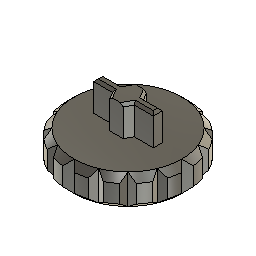
Better screw tool v4 (Autodesk Fusion 360 design; units mm, degrees)
Autodesk Fusion 360 part; units mm, degrees
note: some values were not read from the file. Set by a fixed rule: which sketch regions a step uses.
sketch "Sketch2" plane through (0, 0, 0) normal (0, 0, 1) x (1, 0, 0)
  circle A0 centre (0, 0) radius 10
  constraint coincident A0.centre origin
extrude "Extrude1" add sketch "Sketch2" along normal blind 5
chamfer "Chamfer1" distance 1 angle 45 2 edges at (-9.3233, -3.6162, 5) (-9.3233, -3.6162, 0)
sketch "Sketch3" plane through (0, 0, 5) normal (0, 0, 1) x (-1, 0, 0)
  circle A0 centre (0, 0) radius 9
  line L0 (1, -10) -> (0, -9)
  line L1 (1, -10) -> (2.4142, -10) construction
  line L2 (0, -9) -> (-1, -10)
  line L3 (-1, -10) -> (1, -10)
  dimension "d4" = 135
  constraint horizontal L1
  constraint coincident A0 L0.end
  constraint perpendicular L0 L2
  constraint parallel L1 L3
  measures "d4" angle of L0 L1
extrude "Extrude2" cut sketch "Sketch3" against normal blind 5 contours L0 L2 L3
pattern_circular "C-Pattern1" count 16 over 360 about axis through (0, 0, 1.75) along (0, 0, 1) of "Extrude2"
sketch "Sketch4" plane through (0, 0, 5) normal (0, 0, 1) x (-1, 0, 0)
  arc A0 (-3.4442, -8.3149) -> (0, -9) centre (0, 0) ccw
  arc A1 (0, -9) -> (3.4442, -8.3149) centre (0, 0) ccw
  arc A2 (3.4442, -8.3149) -> (6.364, -6.364) centre (0, 0) ccw
  arc A3 (6.364, -6.364) -> (8.3149, -3.4442) centre (0, 0) ccw
  arc A4 (8.3149, -3.4442) -> (9, 0) centre (0, 0) ccw
  arc A5 (9, 0) -> (8.3149, 3.4442) centre (0, 0) ccw
  arc A6 (8.3149, 3.4442) -> (6.364, 6.364) centre (0, 0) ccw
  arc A7 (6.364, 6.364) -> (3.4442, 8.3149) centre (0, 0) ccw
  arc A8 (3.4442, 8.3149) -> (0, 9) centre (0, 0) ccw
  arc A9 (0, 9) -> (-3.4442, 8.3149) centre (0, 0) ccw
  arc A10 (-3.4442, 8.3149) -> (-6.364, 6.364) centre (0, 0) ccw
  arc A11 (-6.364, 6.364) -> (-8.3149, 3.4442) centre (0, 0) ccw
  arc A12 (-8.3149, 3.4442) -> (-9, 0) centre (0, 0) ccw
  arc A13 (-9, 0) -> (-8.3149, -3.4442) centre (0, 0) ccw
  arc A14 (-8.3149, -3.4442) -> (-6.364, -6.364) centre (0, 0) ccw
  arc A15 (-6.364, -6.364) -> (-3.4442, -8.3149) centre (0, 0) ccw
  line L0 (5, 0.75) -> (-5, 0.75)
  line L1 (-5, 0.75) -> (-5, -0.75)
  line L2 (-5, -0.75) -> (5, -0.75)
  line L3 (5, -0.75) -> (5, 0.75)
  line L4 (5, 0.75) -> (-5, -0.75) construction
  line L5 (-5, 0.75) -> (5, -0.75) construction
  line L6 (-1.1258, -1.95) -> (1.1258, -1.95)
  line L7 (1.1258, -1.95) -> (2.2517, 0)
  line L8 (2.2517, 0) -> (1.1258, 1.95)
  line L9 (1.1258, 1.95) -> (-1.1258, 1.95)
  line L10 (-1.1258, 1.95) -> (-2.2517, 0)
  line L11 (-2.2517, 0) -> (-1.1258, -1.95)
  dimension "d9" = 10
  dimension "d10" = 1.5
  dimension "d11" = 1.95
  constraint perpendicular L0 L1
  constraint parallel L0 L2
  constraint parallel L1 L3
  constraint horizontal L0
  constraint coincident L4 A0.centre
  constraint coincident L5 A0.centre
  constraint coincident A0.centre A1.centre
  constraint parallel L2 L6
  measures "d9" distance of L1.end L2.end
  measures "d10" distance of L0.end L1.end
  measures "d11" distance of A0.centre L11
extrude "Extrude3" add sketch "Sketch4" along normal blind 5 contours L0 L2 L3 L7 L8 | L0 L2 L7 L8 L10 L11 | L0 L8 L9 L10 | L0 L1 L2 L10 L11 | L2 L6 L7 L11
chamfer "Chamfer2" distance 0.4 angle 45 8 edges at (1.4722, -1.35, 10) (1.4722, 1.35, 10) (-1.4722, 1.35, 10) (-1.4722, -1.35, 10) (-3.4093, 0.75, 10) (-3.4093, -0.75, 10) (3.4093, -0.75, 10) (3.4093, 0.75, 10)
chamfer "Chamfer3" distance 0.4 angle 45 2 edges at (-5, 0, 10) (5, 0, 10)
